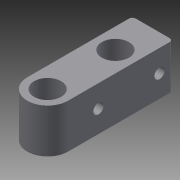
# Autodesk Inventor part: z axis arm3
Saved by Autodesk Inventor 2013 (Build 170138000, 138)
## iProperties
Created: 2017-03-09
Part Number: z axis arm3
Material: Generic
Document SubType Name: Modeling
Designer: Herman de Vries
Density: 1 g/cm^3
Author: Herman de Vries
Autodesk Inventor part; units mm, degrees
ref_plane "YZ Plane" through (0, 0, 0) normal (1, 0, 0) x (0, 1, 0)
ref_plane "XZ Plane" through (0, 0, 0) normal (0, 1, 0) x (-1, 0, 0)
ref_plane "XY Plane" through (0, 0, 0) normal (0, 0, 1) x (1, 0, 0)
sketch "Sketch1" plane through (0, 0, 0) normal (0, 0, 1) x (1, 0, 0)
  line L0 (0, 0) -> (12, 0) construction
  line L1 (12, 0) -> (12, 25)
  line L2 (12, 25) -> (0, 25) construction
  line L3 (0, 25) -> (0, 0)
  arc A0 (12, 25) -> (0, 25) centre (6, 25) ccw
  arc A1 (0, 0) -> (12, 0) centre (6, 0) ccw
  circle A2 centre (6, 0) radius 4
  circle A3 centre (6, 20) radius 4
  line L4 (0, 25) -> (12, 25)
  line L5 (12, 25) -> (12, 31)
  line L6 (12, 31) -> (0, 31)
  line L7 (0, 31) -> (0, 25)
  dimension "d0" = 12
  dimension "d1" = 25
  dimension "d3" = 8
  dimension "d16" = 8
  dimension "d17" = 20
  constraints: 16 end point, 4 centre point, 4 parallel, 4 point on circle, 2 horizontal, 2 midpoint, 2 perpendicular, 1 coincident, 1 collinear, 1 tangent, 1 vertical alignment
  measures "d0" distance of L2.end L1.end
  measures "d1" distance of L1.end L0.end
  measures "d3" diameter of A2
  measures "d16" diameter of A3
  measures "d17" distance of A3.centre A1.centre
extrude "Extrusion1" add sketch "Sketch1" along normal blind 13
sketch "Sketch2" plane through (12, 0, 0) normal (1, 0, 0) x (0, 0, -1)
  circle A0 centre (-6.5, 27) radius 1.5
  circle A1 centre (-6.5, 9) radius 1.5
  line L0 (0, 0) -> (-13, 0) projected
  point P0 (-6.5, 0)
  dimension "d6" = 3
  dimension "d7" = 3
  dimension "d8" = 18
  dimension "d9" = 9
  constraints: 2 centre point, 2 vertical alignment, 1 midpoint
  measures "d6" diameter of A0
  measures "d7" diameter of A1
  measures "d8" distance of A0.centre A1.centre
  measures "d9" distance from line of L0 A1.centre
extrude "Extrusion2" cut sketch "Sketch2" against normal through all
sketch "Sketch3" plane through (0, 0, 0) normal (-1, 0, 0) x (0, 0, 1)
  circle A0 centre (6.5, 27) radius 1.5 projected
  circle A1 centre (6.5, 9) radius 1.5 projected
  circle A2 centre (6.5, 27) radius 3
  circle A3 centre (6.5, 9) radius 3
  point P0 (0, 0)
  dimension "d12" = 6
  dimension "d13" = 6
  constraints: 2 centre point, 2 coincident
  measures "d12" diameter of A2
  measures "d13" diameter of A3
extrude "Extrusion3" cut sketch "Sketch3" against normal blind 3
fillet "Fillet1" radius 1 2 edges at (0, 31, 6.5) (12, 31, 6.5)
body "Solid1"
